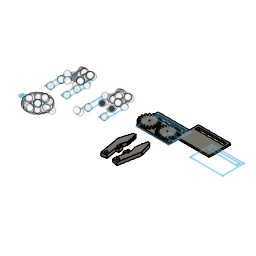
Garra-GSMAKERLAB (Autodesk Fusion 360 design; units mm, degrees)
part number: 2026-05-25-20-05-07-286
Autodesk Fusion 360 part; units mm, degrees
(part 1 of 2)
sketch "Esboço1" plane through (0, 0, 0) normal (0, 1, 0) x (1, 0, 0)
  line L0 (16, 125) -> (21, 125)
  line L1 (21, 103) -> (11, 103)
  line L2 (11, 103) -> (11, 125)
  line L3 (25, 125) -> (30, 125)
  line L4 (35, 125) -> (35, 103)
  line L5 (30, 103) -> (25, 103)
  line L6 (16, 108.5) -> (16, 125) construction
  line L7 (16, 114) -> (21, 114) construction
  line L8 (16, 114) -> (21, 114)
  line L9 (16, 119.5) -> (16, 125) construction
  line L10 (11, 119.5) -> (10, 119.5) construction
  line L11 (10, 119.5) -> (11, 119.5) construction
  line L12 (16, 119.5) -> (21, 119.5) construction
  line L13 (16, 103) -> (16, 114) construction
  line L14 (16, 108.5) -> (21, 108.5) construction
  line L15 (16, 108.5) -> (21, 108.5)
  line L16 (16, 108.5) -> (16, 114)
  line L17 (16, 119.5) -> (21, 119.5)
  line L18 (16, 119.5) -> (16, 125)
  line L19 (25, 114) -> (30, 114) construction
  line L20 (25, 114) -> (30, 114)
  line L21 (25, 119.5) -> (25, 125) construction
  line L22 (25, 119.5) -> (30, 119.5) construction
  line L23 (25, 114) -> (25, 108.5) construction
  line L24 (25, 108.5) -> (30, 108.5) construction
  line L25 (25, 108.5) -> (30, 108.5) construction
  line L26 (25, 108.5) -> (30, 108.5)
  line L27 (25, 119.5) -> (30, 119.5)
  line L28 (25, 108.5) -> (25, 114)
  line L29 (25, 119.5) -> (25, 125)
  line L30 (21, 119.5) -> (21, 114)
  line L31 (11, 103) -> (11, 100)
  line L32 (11, 100) -> (16, 100)
  line L33 (25, 103) -> (25, 100)
  line L34 (25, 100) -> (35, 100)
  line L35 (35, 100) -> (35, 103)
  line L36 (11, 125) -> (11, 127)
  line L37 (11, 127) -> (21, 127)
  line L38 (21, 127) -> (21, 125)
  line L39 (30, 127) -> (35, 127)
  line L40 (35, 125) -> (35, 127)
  line L41 (21, 108.5) -> (21, 103)
  line L42 (16, 103) -> (16, 100)
  line L43 (30, 125) -> (30, 127)
  line L44 (30, 103) -> (30, 108.5)
  line L45 (30, 114) -> (30, 119.5)
  arc A0 (237.1086, 129.0251) -> (213.2904, 133.6785) centre (216.5857, 87.2619) ccw
  arc A1 (237.2082, 125) -> (237.1086, 129.0251) centre (155.7746, 125) ccw
  arc A2 (213.2904, 116.3215) -> (237.1086, 120.9749) centre (216.5857, 162.7381) ccw
  arc A3 (237.1086, 120.9749) -> (237.2082, 125) centre (155.7746, 125) ccw
  arc A4 (230.8269, 156.6003) -> (206.8535, 152.8267) centre (225.8255, 110.3364) ccw
  arc A5 (212.79, 136.5164) -> (233.5803, 149.0355) centre (200.0111, 181.2609) ccw
  arc A6 (233.5803, 149.0355) -> (232.2971, 152.8519) centre (155.7746, 125) ccw
  arc A7 (232.2971, 152.8519) -> (230.8269, 156.6003) centre (155.7746, 125) ccw
  arc A8 (215.4928, 180.3639) -> (194.2558, 168.6185) centre (226.6162, 135.1795) ccw
  arc A9 (205.4127, 155.3223) -> (220.6674, 174.1971) centre (178.101, 192.9977) ccw
  arc A10 (220.6674, 174.1971) -> (218.1563, 177.3445) centre (155.7746, 125) ccw
  arc A11 (218.1563, 177.3445) -> (215.4928, 180.3639) centre (155.7746, 125) ccw
  arc A12 (192.9557, 197.4499) -> (177.0167, 179.1494) centre (218.8623, 158.7949) ccw
  arc A13 (192.0483, 170.4709) -> (199.9275, 193.4248) centre (153.4979, 196.533) ccw
  arc A14 (199.9275, 193.4248) -> (196.4914, 195.5235) centre (155.7746, 125) ccw
  arc A15 (196.4914, 195.5235) -> (192.9557, 197.4499) centre (155.7746, 125) ccw
  arc A16 (165.9341, 205.7973) -> (157.2155, 183.149) centre (203.4991, 178.3341) ccw
  arc A17 (174.3087, 180.135) -> (173.8621, 204.3994) centre (129.1695, 191.4404) ccw
  arc A18 (173.8621, 204.3994) -> (169.9154, 205.1964) centre (155.7746, 125) ccw
  arc A19 (169.9154, 205.1964) -> (165.9341, 205.7973) centre (155.7746, 125) ccw
  arc A20 (137.6871, 204.3994) -> (137.2404, 180.135) centre (182.3797, 191.4404) ccw
  arc A21 (154.3337, 183.149) -> (145.6151, 205.7973) centre (108.05, 178.3341) ccw
  arc A22 (145.6151, 205.7973) -> (141.6338, 205.1964) centre (155.7746, 125) ccw
  arc A23 (141.6338, 205.1964) -> (137.6871, 204.3994) centre (155.7746, 125) ccw
  arc A24 (111.6217, 193.4248) -> (119.5009, 170.4709) centre (158.0512, 196.533) ccw
  arc A25 (134.5325, 179.1494) -> (118.5935, 197.4499) centre (92.6869, 158.7949) ccw
  arc A26 (118.5935, 197.4499) -> (115.0578, 195.5235) centre (155.7746, 125) ccw
  arc A27 (115.0578, 195.5235) -> (111.6217, 193.4248) centre (155.7746, 125) ccw
  arc A28 (90.8818, 174.1971) -> (106.1365, 155.3223) centre (133.4482, 192.9977) ccw
  arc A29 (117.2934, 168.6185) -> (96.0564, 180.3639) centre (84.933, 135.1795) ccw
  arc A30 (96.0564, 180.3639) -> (93.3929, 177.3445) centre (155.7746, 125) ccw
  arc A31 (93.3929, 177.3445) -> (90.8818, 174.1971) centre (155.7746, 125) ccw
  arc A32 (77.9689, 149.0355) -> (98.7592, 136.5164) centre (111.5381, 181.2609) ccw
  arc A33 (104.6957, 152.8267) -> (80.7223, 156.6003) centre (85.7237, 110.3364) ccw
  arc A34 (80.7223, 156.6003) -> (79.2521, 152.8519) centre (155.7746, 125) ccw
  arc A35 (79.2521, 152.8519) -> (77.9689, 149.0355) centre (155.7746, 125) ccw
  arc A36 (74.4406, 120.9749) -> (98.2588, 116.3215) centre (94.9635, 162.7381) ccw
  arc A37 (98.2588, 133.6785) -> (74.4406, 129.0251) centre (94.9635, 87.2619) ccw
  arc A38 (74.4406, 129.0251) -> (74.341, 125) centre (155.7746, 125) ccw
  arc A39 (74.341, 125) -> (74.4406, 120.9749) centre (155.7746, 125) ccw
  arc A40 (80.7223, 93.3997) -> (104.6957, 97.1733) centre (85.7237, 139.6636) ccw
  arc A41 (98.7592, 113.4836) -> (77.9689, 100.9645) centre (111.5381, 68.7391) ccw
  arc A42 (77.9689, 100.9645) -> (79.2521, 97.1481) centre (155.7746, 125) ccw
  arc A43 (79.2521, 97.1481) -> (80.7223, 93.3997) centre (155.7746, 125) ccw
  arc A44 (96.0564, 69.6361) -> (117.2934, 81.3815) centre (84.933, 114.8205) ccw
  arc A45 (106.1365, 94.6777) -> (90.8818, 75.8029) centre (133.4482, 57.0023) ccw
  arc A46 (90.8818, 75.8029) -> (93.3929, 72.6555) centre (155.7746, 125) ccw
  arc A47 (93.3929, 72.6555) -> (96.0564, 69.6361) centre (155.7746, 125) ccw
  arc A48 (118.5935, 52.5501) -> (134.5325, 70.8506) centre (92.6869, 91.2051) ccw
  arc A49 (119.5009, 79.5291) -> (111.6217, 56.5752) centre (158.0512, 53.467) ccw
  arc A50 (111.6217, 56.5752) -> (115.0578, 54.4765) centre (155.7746, 125) ccw
  arc A51 (115.0578, 54.4765) -> (118.5935, 52.5501) centre (155.7746, 125) ccw
  arc A52 (145.6151, 44.2027) -> (154.3337, 66.851) centre (108.05, 71.6659) ccw
  arc A53 (137.2404, 69.865) -> (137.6871, 45.6006) centre (182.3797, 58.5596) ccw
  arc A54 (137.6871, 45.6006) -> (141.6338, 44.8036) centre (155.7746, 125) ccw
  arc A55 (141.6338, 44.8036) -> (145.6151, 44.2027) centre (155.7746, 125) ccw
  arc A56 (173.8621, 45.6006) -> (174.3087, 69.865) centre (129.1695, 58.5596) ccw
  arc A57 (157.2155, 66.851) -> (165.9341, 44.2027) centre (203.4991, 71.6659) ccw
  arc A58 (165.9341, 44.2027) -> (169.9154, 44.8036) centre (155.7746, 125) ccw
  arc A59 (169.9154, 44.8036) -> (173.8621, 45.6006) centre (155.7746, 125) ccw
  arc A60 (199.9275, 56.5752) -> (192.0483, 79.5291) centre (153.4979, 53.467) ccw
  arc A61 (177.0167, 70.8506) -> (192.9557, 52.5501) centre (218.8623, 91.2051) ccw
  arc A62 (192.9557, 52.5501) -> (196.4914, 54.4765) centre (155.7746, 125) ccw
  arc A63 (196.4914, 54.4765) -> (199.9275, 56.5752) centre (155.7746, 125) ccw
  arc A64 (220.6674, 75.8029) -> (205.4127, 94.6777) centre (178.101, 57.0023) ccw
  arc A65 (194.2558, 81.3815) -> (215.4928, 69.6361) centre (226.6162, 114.8205) ccw
  arc A66 (215.4928, 69.6361) -> (218.1563, 72.6555) centre (155.7746, 125) ccw
  arc A67 (218.1563, 72.6555) -> (220.6674, 75.8029) centre (155.7746, 125) ccw
  arc A68 (233.5803, 100.9645) -> (212.79, 113.4836) centre (200.0111, 68.7391) ccw
  arc A69 (206.8535, 97.1733) -> (230.8269, 93.3997) centre (225.8255, 139.6636) ccw
  arc A70 (230.8269, 93.3997) -> (232.2971, 97.1481) centre (155.7746, 125) ccw
  arc A71 (232.2971, 97.1481) -> (233.5803, 100.9645) centre (155.7746, 125) ccw
  arc A72 (106.1365, 155.3223) -> (104.6957, 152.8267) centre (155.7746, 125) ccw
  arc A73 (119.5009, 170.4709) -> (117.2934, 168.6185) centre (155.7746, 125) ccw
  arc A74 (137.2404, 180.135) -> (134.5325, 179.1494) centre (155.7746, 125) ccw
  arc A75 (157.2155, 183.149) -> (154.3337, 183.149) centre (155.7746, 125) ccw
  arc A76 (177.0167, 179.1494) -> (174.3087, 180.135) centre (155.7746, 125) ccw
  arc A77 (194.2558, 168.6185) -> (192.0483, 170.4709) centre (155.7746, 125) ccw
  arc A78 (206.8535, 152.8267) -> (205.4127, 155.3223) centre (155.7746, 125) ccw
  arc A79 (213.2904, 133.6785) -> (212.79, 136.5164) centre (155.7746, 125) ccw
  arc A80 (212.79, 113.4836) -> (213.2904, 116.3215) centre (155.7746, 125) ccw
  arc A81 (205.4127, 94.6777) -> (206.8535, 97.1733) centre (155.7746, 125) ccw
  arc A82 (192.0483, 79.5291) -> (194.2558, 81.3815) centre (155.7746, 125) ccw
  arc A83 (174.3087, 69.865) -> (177.0167, 70.8506) centre (155.7746, 125) ccw
  arc A84 (154.3337, 66.851) -> (157.2155, 66.851) centre (155.7746, 125) ccw
  arc A85 (134.5325, 70.8506) -> (137.2404, 69.865) centre (155.7746, 125) ccw
  arc A86 (117.2934, 81.3815) -> (119.5009, 79.5291) centre (155.7746, 125) ccw
  arc A87 (104.6957, 97.1733) -> (106.1365, 94.6777) centre (155.7746, 125) ccw
  arc A88 (98.7592, 136.5164) -> (98.2588, 133.6785) centre (155.7746, 125) ccw
  arc A89 (98.2588, 116.3215) -> (98.7592, 113.4836) centre (155.7746, 125) ccw
  circle A90 centre (155.7746, 125) radius 5.4289
  line L46 (120, 600) -> (106.1803, 600)
  arc A91 (106.1803, 600) -> (96.5303, 592.6223) centre (106.1803, 590) ccw
  circle A92 centre (75, 425) radius 12.5
  line L47 (50, 497.6393) -> (50, 450)
  line L48 (50, 450) -> (50, 400)
  line L49 (101.0557, 452.1115) -> (123.4164, 496.8328)
  arc A93 (51.0557, 502.1115) -> (50, 497.6393) centre (60, 497.6393) ccw
  arc A94 (106.1803, 600) -> (97.2361, 594.4721) centre (106.1803, 590) ccw
  line L50 (51.0557, 502.1115) -> (97.2361, 594.4721)
  arc A95 (123.4164, 496.8328) -> (124.5987, 500.0947) centre (110, 503.541) ccw
  line L51 (100, 400) -> (100, 447.6393)
  arc A96 (101.0557, 452.1115) -> (100, 447.6393) centre (110, 447.6393) ccw
  line L52 (120, 600) -> (106.1803, 600)
  circle A97 centre (75, 425) radius 12.5
  line L53 (250, 400) -> (250, 497.732)
  line L54 (200, 400) -> (200, 446.5033)
  line L55 (198.9884, 450.8862) -> (176.5174, 496.9698)
  line L56 (180, 600) -> (196.9111, 600)
  line L57 (201.3824, 597.2378) -> (248.9426, 502.2076)
  arc A98 (200, 446.5033) -> (198.9884, 450.8862) centre (190, 446.5033) ccw
  arc A99 (175.3938, 500.1297) -> (176.5174, 496.9698) centre (190, 503.544) ccw
  arc A100 (180, 600) -> (175.3489, 596.8351) centre (180, 595) ccw
  arc A101 (124.6389, 596.8655) -> (120, 600) centre (120, 595) ccw
  arc A102 (201.3824, 597.2378) -> (196.9111, 600) centre (196.9111, 595) ccw
  arc A103 (250, 497.732) -> (248.9426, 502.2076) centre (240, 497.732) ccw
  circle A104 centre (225, 423.2517) radius 12.5
  arc A105 (125, 510.1754) -> (125, 505.1805) centre (124.8879, 507.678) ccw
  line L58 (125, 505.0754) -> (125, 505.1805)
  line L59 (125, 505.0754) -> (125, 505.1805)
  arc A106 (125, 520.3754) -> (125, 515.3805) centre (124.8879, 517.878) ccw
  arc A107 (125, 530.5754) -> (125, 525.5805) centre (124.8879, 528.078) ccw
  arc A108 (125, 540.7754) -> (125, 535.7805) centre (124.8879, 538.278) ccw
  arc A109 (125, 550.9754) -> (125, 545.9805) centre (124.8879, 548.478) ccw
  arc A110 (125, 561.1754) -> (125, 556.1805) centre (124.8879, 558.678) ccw
  arc A111 (125, 571.3754) -> (125, 566.3805) centre (124.8879, 568.878) ccw
  arc A112 (125, 581.5754) -> (125, 576.5805) centre (124.8879, 579.078) ccw
  arc A113 (125, 591.7754) -> (125, 586.7805) centre (124.8879, 589.278) ccw
  line L60 (125, 591.7754) -> (125, 591.8805)
  line L61 (125, 591.7754) -> (125, 591.8805)
  arc A114 (175, 510.2805) -> (175, 515.2754) centre (174.8879, 512.778) ccw
  arc A115 (175, 520.4805) -> (175, 525.4754) centre (174.8879, 522.978) ccw
  arc A116 (175, 530.6805) -> (175, 535.6754) centre (174.8879, 533.178) ccw
  arc A117 (175, 540.8805) -> (175, 545.8754) centre (174.8879, 543.378) ccw
  arc A118 (175, 551.0805) -> (175, 556.0754) centre (174.8879, 553.578) ccw
  arc A119 (175, 561.2805) -> (175, 566.2754) centre (174.8879, 563.778) ccw
  arc A120 (175, 571.4805) -> (175, 576.4754) centre (174.8879, 573.978) ccw
  arc A121 (175, 581.6805) -> (175, 586.6754) centre (174.8879, 584.178) ccw
  arc A122 (175, 591.8805) -> (175.3489, 596.8351) centre (174.8879, 594.378) ccw
  arc A123 (124.5987, 500.0947) -> (125, 505.0754) centre (124.8879, 502.578) ccw
  arc A124 (125, 510.2805) -> (125, 515.2754) centre (124.8879, 512.778) ccw
  line L62 (125, 510.1754) -> (125, 510.2805)
  line L63 (125, 515.2754) -> (125, 515.3805)
  line L64 (125, 510.1754) -> (125, 510.2805)
  line L65 (125, 515.2754) -> (125, 515.3805)
  arc A125 (125, 520.4805) -> (125, 525.4754) centre (124.8879, 522.978) ccw
  line L66 (125, 520.3754) -> (125, 520.4805)
  line L67 (125, 525.4754) -> (125, 525.5805)
  line L68 (125, 520.3754) -> (125, 520.4805)
  line L69 (125, 525.4754) -> (125, 525.5805)
  arc A126 (125, 530.6805) -> (125, 535.6754) centre (124.8879, 533.178) ccw
  line L70 (125, 530.5754) -> (125, 530.6805)
  line L71 (125, 535.6754) -> (125, 535.7805)
  line L72 (125, 530.5754) -> (125, 530.6805)
  line L73 (125, 535.6754) -> (125, 535.7805)
  arc A127 (125, 540.8805) -> (125, 545.8754) centre (124.8879, 543.378) ccw
  line L74 (125, 540.7754) -> (125, 540.8805)
  line L75 (125, 545.8754) -> (125, 545.9805)
  line L76 (125, 540.7754) -> (125, 540.8805)
  line L77 (125, 545.8754) -> (125, 545.9805)
  arc A128 (125, 551.0805) -> (125, 556.0754) centre (124.8879, 553.578) ccw
  line L78 (125, 550.9754) -> (125, 551.0805)
  line L79 (125, 556.0754) -> (125, 556.1805)
  line L80 (125, 550.9754) -> (125, 551.0805)
  line L81 (125, 556.0754) -> (125, 556.1805)
  arc A129 (125, 561.2805) -> (125, 566.2754) centre (124.8879, 563.778) ccw
  line L82 (125, 561.1754) -> (125, 561.2805)
  line L83 (125, 566.2754) -> (125, 566.3805)
  line L84 (125, 561.1754) -> (125, 561.2805)
  line L85 (125, 566.2754) -> (125, 566.3805)
  arc A130 (125, 571.4805) -> (125, 576.4754) centre (124.8879, 573.978) ccw
  line L86 (125, 571.3754) -> (125, 571.4805)
  line L87 (125, 576.4754) -> (125, 576.5805)
  line L88 (125, 571.3754) -> (125, 571.4805)
  line L89 (125, 576.4754) -> (125, 576.5805)
  arc A131 (125, 581.6805) -> (125, 586.6754) centre (124.8879, 584.178) ccw
  line L90 (125, 581.5754) -> (125, 581.6805)
  line L91 (125, 586.6754) -> (125, 586.7805)
  line L92 (125, 581.5754) -> (125, 581.6805)
  line L93 (125, 586.6754) -> (125, 586.7805)
  arc A132 (125, 591.8805) -> (124.6389, 596.8655) centre (124.8879, 594.378) ccw
  arc A133 (175, 510.1754) -> (175, 505.1805) centre (174.8879, 507.678) ccw
  line L94 (175, 505.0754) -> (175, 505.1805)
  line L95 (175, 510.1754) -> (175, 510.2805)
  arc A134 (175, 520.3754) -> (175, 515.3805) centre (174.8879, 517.878) ccw
  line L96 (175, 515.2754) -> (175, 515.3805)
  line L97 (175, 520.3754) -> (175, 520.4805)
  arc A135 (175, 530.5754) -> (175, 525.5805) centre (174.8879, 528.078) ccw
  line L98 (175, 525.4754) -> (175, 525.5805)
  line L99 (175, 530.5754) -> (175, 530.6805)
  arc A136 (175, 540.7754) -> (175, 535.7805) centre (174.8879, 538.278) ccw
  line L100 (175, 535.6754) -> (175, 535.7805)
  line L101 (175, 540.7754) -> (175, 540.8805)
  arc A137 (175, 550.9754) -> (175, 545.9805) centre (174.8879, 548.478) ccw
  line L102 (175, 545.8754) -> (175, 545.9805)
  line L103 (175, 550.9754) -> (175, 551.0805)
  arc A138 (175, 561.1754) -> (175, 556.1805) centre (174.8879, 558.678) ccw
  line L104 (175, 556.0754) -> (175, 556.1805)
  line L105 (175, 561.1754) -> (175, 561.2805)
  arc A139 (175, 571.3754) -> (175, 566.3805) centre (174.8879, 568.878) ccw
  line L106 (175, 566.2754) -> (175, 566.3805)
  line L107 (175, 571.3754) -> (175, 571.4805)
  arc A140 (175, 581.5754) -> (175, 576.5805) centre (174.8879, 579.078) ccw
  line L108 (175, 576.4754) -> (175, 576.5805)
  line L109 (175, 581.5754) -> (175, 581.6805)
  arc A141 (175, 591.7754) -> (175, 586.7805) centre (174.8879, 589.278) ccw
  line L110 (175, 586.6754) -> (175, 586.7805)
  line L111 (175, 591.7754) -> (175, 591.8805)
  arc A142 (175.3938, 500.1297) -> (175, 505.0754) centre (174.8879, 502.578) ccw
  line L112 (50, 400) -> (50, 300)
  line L113 (50, 300) -> (100, 300)
  line L114 (100, 300) -> (100, 400)
  line L115 (200, 400) -> (200, 300)
  line L116 (200, 300) -> (250, 300)
  line L117 (250, 300) -> (250, 400)
  circle A143 centre (75, 325) radius 12.5
  circle A144 centre (225, 325) radius 12.5
  circle A145 centre (251, 128) radius 7.2111
  circle A146 centre (281, 133) radius 10.5
  line L118 (100, 300) -> (125, 300) construction
  line L119 (125, 300) -> (125, 250) construction
  line L120 (125, 250) -> (45, 250) construction
  line L121 (45, 250) -> (45, 300) construction
  line L122 (45, 300) -> (50, 300) construction
  line L123 (100, 300) -> (125, 250) construction
  line L124 (50, 300) -> (75, 250) construction
  line L125 (800, 600) -> (1100, 600)
  line L126 (1100, 600) -> (1100, 400)
  line L127 (1100, 400) -> (800, 400)
  line L128 (800, 400) -> (800, 600)
  line L129 (1000, 500) -> (1090, 500)
  line L130 (1090, 500) -> (1090, 450)
  line L131 (1090, 450) -> (1000, 450)
  line L132 (1000, 450) -> (1000, 500)
  line L133 (820, 580) -> (1080, 580)
  line L134 (1080, 580) -> (1080, 550)
  line L135 (1080, 550) -> (820, 550)
  line L136 (820, 550) -> (820, 580)
  arc A147 (104.6957, 152.8267) -> (80.7223, 156.6003) centre (85.7237, 110.3364) ccw
  arc A148 (232.2971, 152.8519) -> (230.8269, 156.6003) centre (155.7746, 125) ccw
  arc A149 (141.6338, 205.1964) -> (137.6871, 204.3994) centre (155.7746, 125) ccw
  arc A150 (206.8535, 152.8267) -> (205.4127, 155.3223) centre (155.7746, 125) ccw
  arc A151 (230.8269, 156.6003) -> (206.8535, 152.8267) centre (225.8255, 110.3364) ccw
  arc A152 (80.7223, 156.6003) -> (79.2521, 152.8519) centre (155.7746, 125) ccw
  arc A153 (154.3337, 183.149) -> (145.6151, 205.7973) centre (108.05, 178.3341) ccw
  arc A154 (145.6151, 205.7973) -> (141.6338, 205.1964) centre (155.7746, 125) ccw
  arc A155 (137.6871, 204.3994) -> (137.2404, 180.135) centre (182.3797, 191.4404) ccw
  arc A156 (220.6674, 75.8029) -> (205.4127, 94.6777) centre (178.101, 57.0023) ccw
  arc A157 (194.2558, 81.3815) -> (215.4928, 69.6361) centre (226.6162, 114.8205) ccw
  arc A158 (104.6957, 97.1733) -> (106.1365, 94.6777) centre (155.7746, 125) ccw
  arc A159 (169.9154, 44.8036) -> (173.8621, 45.6006) centre (155.7746, 125) ccw
  arc A160 (232.2971, 97.1481) -> (233.5803, 100.9645) centre (155.7746, 125) ccw
  arc A161 (118.5935, 52.5501) -> (134.5325, 70.8506) centre (92.6869, 91.2051) ccw
  arc A162 (90.8818, 75.8029) -> (93.3929, 72.6555) centre (155.7746, 125) ccw
  arc A163 (218.1563, 72.6555) -> (220.6674, 75.8029) centre (155.7746, 125) ccw
  arc A164 (174.3087, 69.865) -> (177.0167, 70.8506) centre (155.7746, 125) ccw
  arc A165 (206.8535, 97.1733) -> (230.8269, 93.3997) centre (225.8255, 139.6636) ccw
  arc A166 (137.6871, 45.6006) -> (141.6338, 44.8036) centre (155.7746, 125) ccw
  arc A167 (165.9341, 44.2027) -> (169.9154, 44.8036) centre (155.7746, 125) ccw
  arc A168 (137.2404, 69.865) -> (137.6871, 45.6006) centre (182.3797, 58.5596) ccw
  arc A169 (111.6217, 56.5752) -> (115.0578, 54.4765) centre (155.7746, 125) ccw
  arc A170 (117.2934, 81.3815) -> (119.5009, 79.5291) centre (155.7746, 125) ccw
  arc A171 (145.6151, 44.2027) -> (154.3337, 66.851) centre (108.05, 71.6659) ccw
  arc A172 (93.3929, 72.6555) -> (96.0564, 69.6361) centre (155.7746, 125) ccw
  arc A173 (134.5325, 70.8506) -> (137.2404, 69.865) centre (155.7746, 125) ccw
  arc A174 (215.4928, 69.6361) -> (218.1563, 72.6555) centre (155.7746, 125) ccw
  arc A175 (199.9275, 56.5752) -> (192.0483, 79.5291) centre (153.4979, 53.467) ccw
  arc A176 (173.8621, 45.6006) -> (174.3087, 69.865) centre (129.1695, 58.5596) ccw
  arc A177 (141.6338, 44.8036) -> (145.6151, 44.2027) centre (155.7746, 125) ccw
  arc A178 (192.9557, 52.5501) -> (196.4914, 54.4765) centre (155.7746, 125) ccw
  arc A179 (106.1365, 94.6777) -> (90.8818, 75.8029) centre (133.4482, 57.0023) ccw
  arc A180 (230.8269, 93.3997) -> (232.2971, 97.1481) centre (155.7746, 125) ccw
  arc A181 (196.4914, 54.4765) -> (199.9275, 56.5752) centre (155.7746, 125) ccw
  arc A182 (177.0167, 70.8506) -> (192.9557, 52.5501) centre (218.8623, 91.2051) ccw
  arc A183 (192.0483, 79.5291) -> (194.2558, 81.3815) centre (155.7746, 125) ccw
  arc A184 (119.5009, 79.5291) -> (111.6217, 56.5752) centre (158.0512, 53.467) ccw
  arc A185 (117.2934, 168.6185) -> (96.0564, 180.3639) centre (84.933, 135.1795) ccw
  arc A186 (115.0578, 195.5235) -> (111.6217, 193.4248) centre (155.7746, 125) ccw
  arc A187 (111.6217, 193.4248) -> (119.5009, 170.4709) centre (158.0512, 196.533) ccw
  arc A188 (137.2404, 180.135) -> (134.5325, 179.1494) centre (155.7746, 125) ccw
  arc A189 (218.1563, 177.3445) -> (215.4928, 180.3639) centre (155.7746, 125) ccw
  circle A190 centre (155.7746, 125) radius 5.4289
  arc A191 (174.3087, 180.135) -> (173.8621, 204.3994) centre (129.1695, 191.4404) ccw
  arc A192 (77.9689, 149.0355) -> (98.7592, 136.5164) centre (111.5381, 181.2609) ccw
  arc A193 (74.4406, 120.9749) -> (98.2588, 116.3215) centre (94.9635, 162.7381) ccw
  arc A194 (192.0483, 170.4709) -> (199.9275, 193.4248) centre (153.4979, 196.533) ccw
  arc A195 (74.4406, 129.0251) -> (74.341, 125) centre (155.7746, 125) ccw
  arc A196 (74.341, 125) -> (74.4406, 120.9749) centre (155.7746, 125) ccw
  arc A197 (205.4127, 155.3223) -> (220.6674, 174.1971) centre (178.101, 192.9977) ccw
  arc A198 (199.9275, 193.4248) -> (196.4914, 195.5235) centre (155.7746, 125) ccw
  arc A199 (173.8621, 204.3994) -> (169.9154, 205.1964) centre (155.7746, 125) ccw
  arc A200 (79.2521, 152.8519) -> (77.9689, 149.0355) centre (155.7746, 125) ccw
  arc A201 (194.2558, 168.6185) -> (192.0483, 170.4709) centre (155.7746, 125) ccw
  arc A202 (215.4928, 180.3639) -> (194.2558, 168.6185) centre (226.6162, 135.1795) ccw
  arc A203 (233.5803, 149.0355) -> (232.2971, 152.8519) centre (155.7746, 125) ccw
  arc A204 (237.1086, 129.0251) -> (213.2904, 133.6785) centre (216.5857, 87.2619) ccw
  arc A205 (237.2082, 125) -> (237.1086, 129.0251) centre (155.7746, 125) ccw
  arc A206 (98.2588, 133.6785) -> (74.4406, 129.0251) centre (94.9635, 87.2619) ccw
  arc A207 (154.3337, 66.851) -> (157.2155, 66.851) centre (155.7746, 125) ccw
  arc A208 (98.7592, 136.5164) -> (98.2588, 133.6785) centre (155.7746, 125) ccw
  arc A209 (213.2904, 133.6785) -> (212.79, 136.5164) centre (155.7746, 125) ccw
  arc A210 (212.79, 136.5164) -> (233.5803, 149.0355) centre (200.0111, 181.2609) ccw
  arc A211 (177.0167, 179.1494) -> (174.3087, 180.135) centre (155.7746, 125) ccw
  arc A212 (212.79, 113.4836) -> (213.2904, 116.3215) centre (155.7746, 125) ccw
  arc A213 (169.9154, 205.1964) -> (165.9341, 205.7973) centre (155.7746, 125) ccw
  arc A214 (196.4914, 195.5235) -> (192.9557, 197.4499) centre (155.7746, 125) ccw
  arc A215 (165.9341, 205.7973) -> (157.2155, 183.149) centre (203.4991, 178.3341) ccw
  arc A216 (213.2904, 116.3215) -> (237.1086, 120.9749) centre (216.5857, 162.7381) ccw
  arc A217 (205.4127, 94.6777) -> (206.8535, 97.1733) centre (155.7746, 125) ccw
  arc A218 (98.2588, 116.3215) -> (98.7592, 113.4836) centre (155.7746, 125) ccw
  arc A219 (98.7592, 113.4836) -> (77.9689, 100.9645) centre (111.5381, 68.7391) ccw
  arc A220 (77.9689, 100.9645) -> (79.2521, 97.1481) centre (155.7746, 125) ccw
  arc A221 (237.1086, 120.9749) -> (237.2082, 125) centre (155.7746, 125) ccw
  arc A222 (80.7223, 93.3997) -> (104.6957, 97.1733) centre (85.7237, 139.6636) ccw
  arc A223 (220.6674, 174.1971) -> (218.1563, 177.3445) centre (155.7746, 125) ccw
  arc A224 (157.2155, 183.149) -> (154.3337, 183.149) centre (155.7746, 125) ccw
  arc A225 (233.5803, 100.9645) -> (212.79, 113.4836) centre (200.0111, 68.7391) ccw
  arc A226 (157.2155, 66.851) -> (165.9341, 44.2027) centre (203.4991, 71.6659) ccw
  arc A227 (192.9557, 197.4499) -> (177.0167, 179.1494) centre (218.8623, 158.7949) ccw
  arc A228 (90.8818, 174.1971) -> (106.1365, 155.3223) centre (133.4482, 192.9977) ccw
  arc A229 (96.0564, 180.3639) -> (93.3929, 177.3445) centre (155.7746, 125) ccw
  arc A230 (106.1365, 155.3223) -> (104.6957, 152.8267) centre (155.7746, 125) ccw
  arc A231 (93.3929, 177.3445) -> (90.8818, 174.1971) centre (155.7746, 125) ccw
  arc A232 (134.5325, 179.1494) -> (118.5935, 197.4499) centre (92.6869, 158.7949) ccw
  arc A233 (118.5935, 197.4499) -> (115.0578, 195.5235) centre (155.7746, 125) ccw
  arc A234 (119.5009, 170.4709) -> (117.2934, 168.6185) centre (155.7746, 125) ccw
  arc A235 (96.0564, 69.6361) -> (117.2934, 81.3815) centre (84.933, 114.8205) ccw
  arc A236 (79.2521, 97.1481) -> (80.7223, 93.3997) centre (155.7746, 125) ccw
  arc A237 (115.0578, 54.4765) -> (118.5935, 52.5501) centre (155.7746, 125) ccw
  line L137 (100, 445) -> (200, 445) construction
  line L138 (100, 400) -> (200, 400) construction
  line L139 (150, 445) -> (150, 400) construction
  line L140 (400, 450) -> (400, 400)
  line L141 (450, 400) -> (550, 400) construction
  line L142 (600, 300) -> (600, 400)
  arc A238 (600, 497.732) -> (598.9426, 502.2076) centre (590, 497.732) ccw
  line L143 (600, 400) -> (600, 497.732)
  arc A239 (525, 581.5754) -> (525, 576.5805) centre (524.8879, 579.078) ccw
  arc A240 (525, 520.3754) -> (525, 515.3805) centre (524.8879, 517.878) ccw
  line L144 (525, 581.5754) -> (525, 581.6805)
  line L145 (525, 576.4754) -> (525, 576.5805)
  arc A241 (401.0557, 502.1115) -> (400, 497.6393) centre (410, 497.6393) ccw
  line L146 (525, 545.8754) -> (525, 545.9805)
  arc A242 (475, 540.7754) -> (475, 535.7805) centre (474.8879, 538.278) ccw
  arc A243 (475, 510.2805) -> (475, 515.2754) centre (474.8879, 512.778) ccw
  arc A244 (530, 600) -> (525.3489, 596.8351) centre (530, 595) ccw
  line L147 (475, 550.9754) -> (475, 551.0805)
  line L148 (525, 510.1754) -> (525, 510.2805)
  arc A245 (525.3938, 500.1297) -> (525, 505.0754) centre (524.8879, 502.578) ccw
  line L149 (525, 520.3754) -> (525, 520.4805)
  arc A246 (475, 520.3754) -> (475, 515.3805) centre (474.8879, 517.878) ccw
  line L150 (475, 505.0754) -> (475, 505.1805)
  arc A247 (525.3938, 500.1297) -> (526.5174, 496.9698) centre (540, 503.544) ccw
  arc A248 (525, 510.1754) -> (525, 505.1805) centre (524.8879, 507.678) ccw
  arc A249 (525, 591.7754) -> (525, 586.7805) centre (524.8879, 589.278) ccw
  line L151 (475, 591.7754) -> (475, 591.8805)
  line L152 (525, 525.4754) -> (525, 525.5805)
  arc A250 (456.1803, 600) -> (447.2361, 594.4721) centre (456.1803, 590) ccw
  line L153 (475, 545.8754) -> (475, 545.9805)
  line L154 (475, 530.5754) -> (475, 530.6805)
  arc A251 (551.3824, 597.2378) -> (546.9111, 600) centre (546.9111, 595) ccw
  line L155 (475, 520.3754) -> (475, 520.4805)
  line L156 (475, 510.1754) -> (475, 510.2805)
  line L157 (525, 535.6754) -> (525, 535.7805)
  arc A252 (525, 540.8805) -> (525, 545.8754) centre (524.8879, 543.378) ccw
  line L158 (475, 571.3754) -> (475, 571.4805)
  line L159 (475, 545.8754) -> (475, 545.9805)
  line L160 (475, 515.2754) -> (475, 515.3805)
  line L161 (401.0557, 502.1115) -> (447.2361, 594.4721)
  line L162 (525, 530.5754) -> (525, 530.6805)
  arc A253 (475, 550.9754) -> (475, 545.9805) centre (474.8879, 548.478) ccw
  arc A254 (475, 510.1754) -> (475, 505.1805) centre (474.8879, 507.678) ccw
  line L163 (475, 535.6754) -> (475, 535.7805)
  arc A255 (525, 581.6805) -> (525, 586.6754) centre (524.8879, 584.178) ccw
  line L164 (525, 540.7754) -> (525, 540.8805)
  line L165 (400, 400) -> (400, 300)
  arc A256 (525, 540.7754) -> (525, 535.7805) centre (524.8879, 538.278) ccw
  line L166 (450, 300) -> (450, 400)
  line L167 (525, 556.0754) -> (525, 556.1805)
  line L168 (450, 300) -> (475, 250) construction
  line L169 (450, 300) -> (475, 300) construction
  line L170 (525, 571.3754) -> (525, 571.4805)
  line L171 (525, 515.2754) -> (525, 515.3805)
  arc A257 (525, 561.1754) -> (525, 556.1805) centre (524.8879, 558.678) ccw
  arc A258 (525, 530.5754) -> (525, 525.5805) centre (524.8879, 528.078) ccw
  line L172 (525, 561.1754) -> (525, 561.2805)
  arc A259 (525, 520.4805) -> (525, 525.4754) centre (524.8879, 522.978) ccw
  line L173 (550, 400) -> (550, 300)
  arc A260 (525, 571.4805) -> (525, 576.4754) centre (524.8879, 573.978) ccw
  arc A261 (525, 510.2805) -> (525, 515.2754) centre (524.8879, 512.778) ccw
  line L174 (470, 600) -> (456.1803, 600)
  arc A262 (456.1803, 600) -> (446.5303, 592.6223) centre (456.1803, 590) ccw
  line L175 (525, 505.0754) -> (525, 505.1805)
  arc A263 (525, 530.6805) -> (525, 535.6754) centre (524.8879, 533.178) ccw
  arc A264 (525, 571.3754) -> (525, 566.3805) centre (524.8879, 568.878) ccw
  arc A265 (525, 551.0805) -> (525, 556.0754) centre (524.8879, 553.578) ccw
  line L176 (525, 550.9754) -> (525, 551.0805)
  line L177 (475, 540.7754) -> (475, 540.8805)
  line L178 (525, 566.2754) -> (525, 566.3805)
  arc A266 (474.5987, 500.0947) -> (475, 505.0754) centre (474.8879, 502.578) ccw
  arc A267 (525, 561.2805) -> (525, 566.2754) centre (524.8879, 563.778) ccw
  arc A268 (475, 540.8805) -> (475, 545.8754) centre (474.8879, 543.378) ccw
  line L179 (475, 581.5754) -> (475, 581.6805)
  circle A269 centre (575, 325) radius 12.5
  line L180 (470, 600) -> (456.1803, 600)
  line L181 (451.0557, 452.1115) -> (473.4164, 496.8328)
  line L182 (550, 300) -> (600, 300)
  line L183 (400, 497.6393) -> (400, 450)
  line L184 (548.9884, 450.8862) -> (526.5174, 496.9698)
  circle A270 centre (425, 325) radius 12.5
  line L185 (450, 445) -> (550, 445) construction
  line L186 (475, 556.0754) -> (475, 556.1805)
  line L187 (475, 530.5754) -> (475, 530.6805)
  arc A271 (475, 581.5754) -> (475, 576.5805) centre (474.8879, 579.078) ccw
  arc A272 (475, 530.6805) -> (475, 535.6754) centre (474.8879, 533.178) ccw
  line L188 (525, 591.7754) -> (525, 591.8805)
  arc A273 (473.4164, 496.8328) -> (474.5987, 500.0947) centre (460, 503.541) ccw
  line L189 (475, 540.7754) -> (475, 540.8805)
  arc A274 (475, 561.1754) -> (475, 556.1805) centre (474.8879, 558.678) ccw
  arc A275 (475, 561.2805) -> (475, 566.2754) centre (474.8879, 563.778) ccw
  line L190 (525, 586.6754) -> (525, 586.7805)
  line L191 (475, 525.4754) -> (475, 525.5805)
  line L192 (475, 550.9754) -> (475, 551.0805)
  line L193 (475, 510.1754) -> (475, 510.2805)
  line L194 (475, 576.4754) -> (475, 576.5805)
  arc A276 (475, 530.5754) -> (475, 525.5805) centre (474.8879, 528.078) ccw
  arc A277 (525, 591.8805) -> (525.3489, 596.8351) centre (524.8879, 594.378) ccw
  arc A278 (475, 571.4805) -> (475, 576.4754) centre (474.8879, 573.978) ccw
  line L195 (530, 600) -> (546.9111, 600)
  line L196 (475, 556.0754) -> (475, 556.1805)
  line L197 (475, 535.6754) -> (475, 535.7805)
  line L198 (475, 515.2754) -> (475, 515.3805)
  line L199 (475, 586.6754) -> (475, 586.7805)
  arc A279 (474.6389, 596.8655) -> (470, 600) centre (470, 595) ccw
  line L200 (475, 591.7754) -> (475, 591.8805)
  line L201 (475, 561.1754) -> (475, 561.2805)
  arc A280 (475, 571.3754) -> (475, 566.3805) centre (474.8879, 568.878) ccw
  arc A281 (475, 591.7754) -> (475, 586.7805) centre (474.8879, 589.278) ccw
  line L202 (475, 561.1754) -> (475, 561.2805)
  line L203 (475, 566.2754) -> (475, 566.3805)
  line L204 (475, 571.3754) -> (475, 571.4805)
  line L205 (475, 520.3754) -> (475, 520.4805)
  line L206 (475, 566.2754) -> (475, 566.3805)
  line L207 (475, 581.5754) -> (475, 581.6805)
  line L208 (475, 586.6754) -> (475, 586.7805)
  line L209 (475, 525.4754) -> (475, 525.5805)
  line L210 (475, 576.4754) -> (475, 576.5805)
  arc A282 (475, 581.6805) -> (475, 586.6754) centre (474.8879, 584.178) ccw
  arc A283 (475, 591.8805) -> (474.6389, 596.8655) centre (474.8879, 594.378) ccw
  arc A284 (475, 520.4805) -> (475, 525.4754) centre (474.8879, 522.978) ccw
  arc A285 (475, 551.0805) -> (475, 556.0754) centre (474.8879, 553.578) ccw
  line L211 (475, 505.0754) -> (475, 505.1805)
  circle A286 centre (545, 423.2517) radius 12.5
  line L212 (551.3824, 597.2378) -> (598.9426, 502.2076)
  line L213 (550, 445) -> (550, 446.5033)
  line L214 (500, 445) -> (500, 400) construction
  line L215 (475, 300) -> (475, 250) construction
  line L216 (395, 250) -> (395, 300) construction
  arc A287 (525, 550.9754) -> (525, 545.9805) centre (524.8879, 548.478) ccw
  line L217 (395, 300) -> (400, 300) construction
  line L218 (400, 300) -> (425, 250) construction
  line L219 (400, 300) -> (450, 300)
  arc A288 (550, 446.5033) -> (548.9884, 450.8862) centre (540, 446.5033) ccw
  arc A289 (451.0557, 452.1115) -> (450, 447.6393) centre (460, 447.6393) ccw
  circle A290 centre (455, 425) radius 12.5
  line L220 (450, 445) -> (450, 447.6393)
  line L221 (450, 400) -> (470, 400)
  line L222 (450, 445) -> (470, 445)
  line L223 (550, 400) -> (530, 400)
  line L224 (550, 445) -> (530, 445)
  line L225 (470, 400) -> (475, 400)
  line L226 (475, 445) -> (475, 400)
  line L227 (475, 445) -> (470, 445)
  line L228 (530, 400) -> (525, 400)
  line L229 (525, 400) -> (525, 445)
  line L230 (530, 445) -> (525, 445)
  line L231 (455, 425) -> (475, 425) construction
  line L232 (545, 423.2517) -> (525, 423.2517) construction
  line L233 (1580, 550) -> (1320, 550)
  line L234 (1300, 400) -> (1300, 600)
  line L235 (1300, 600) -> (1600, 600)
  line L236 (1320, 550) -> (1320, 580)
  line L237 (1320, 580) -> (1580, 580)
  line L238 (1600, 600) -> (1600, 400)
  line L239 (1580, 580) -> (1580, 550)
  line L240 (1600, 400) -> (1300, 400)
  point P0 (175, 595)
  point P1 (175, 503.541)
  point P2 (175, 503.541)
  point P3 (525, 595)
  point P4 (525, 503.541)
  point P5 (525, 503.541)
  dimension "d29" = 360
  dimension "d40" = 10
  dimension "d44" = 25
  dimension "d45" = 10
  dimension "d46" = 10
  dimension "d47" = 10
  dimension "d48" = 15
  dimension "d49" = 25
  dimension "d51" = 10
  dimension "d52" = 15
  dimension "d53" = 5
  dimension "d54" = 5
  dimension "d55" = 5
  dimension "d56" = 10
  dimension "d57" = 25
  dimension "d58" = 5
  dimension "d59" = 5
  dimension "d60" = 5
  dimension "d61" = 5
  dimension "d62" = 5
  dimension "d63" = 5
  dimension "d64" = 5
  dimension "d65" = 5
  dimension "d66" = 5
  dimension "d67" = 5
  dimension "d68" = 5
  dimension "d69" = 5
  dimension "d70" = 5
  dimension "d71" = 5
  dimension "d72" = 5
  dimension "d73" = 5
  dimension "d74" = 5
  dimension "d75" = 5
  dimension "d76" = 5
  dimension "d79" = 5
  dimension "d80" = 5
  dimension "d81" = 5
  dimension "d82" = 5
  dimension "d83" = 5
  dimension "d84" = 5
  dimension "d85" = 5
  dimension "d86" = 5
  dimension "d87" = 5
  dimension "d88" = 5
  dimension "d89" = 5
  dimension "d90" = 5
  dimension "d91" = 5
  dimension "d92" = 5
  dimension "d93" = 5
  dimension "d94" = 5
  dimension "d95" = 5
  dimension "d96" = 5
  dimension "d97" = 5
  dimension "d101" = 25
  dimension "d102" = 25
  dimension "d113" = 25
  dimension "d114" = 21
  dimension "d122" = 300
  dimension "d123" = 200
  dimension "d127" = 360
  dimension "d135" = 10
  dimension "d137" = 10
  dimension "d138" = 10
  dimension "d139" = 10
  dimension "d140" = 15
  dimension "d141" = 25
  dimension "d142" = 10
  dimension "d143" = 15
  dimension "d144" = 5
  dimension "d145" = 5
  dimension "d146" = 5
  dimension "d147" = 10
  dimension "d148" = 25
  dimension "d149" = 5
  dimension "d150" = 5
  dimension "d151" = 5
  dimension "d152" = 5
  dimension "d153" = 5
  dimension "d154" = 5
  dimension "d155" = 5
  dimension "d156" = 5
  dimension "d157" = 5
  dimension "d158" = 5
  dimension "d159" = 5
  dimension "d160" = 5
  dimension "d161" = 5
  dimension "d162" = 5
  dimension "d163" = 5
  dimension "d164" = 5
  dimension "d165" = 5
  dimension "d166" = 5
  dimension "d167" = 5
  dimension "d168" = 5
  dimension "d169" = 5
  dimension "d170" = 5
  dimension "d171" = 5
  dimension "d172" = 5
  dimension "d173" = 5
  dimension "d174" = 5
  dimension "d175" = 5
  dimension "d176" = 5
  dimension "d177" = 5
  dimension "d178" = 5
  dimension "d179" = 5
  dimension "d180" = 5
  dimension "d181" = 5
  dimension "d182" = 5
  dimension "d183" = 5
  dimension "d184" = 5
  dimension "d185" = 5
  dimension "d186" = 5
  dimension "d187" = 25
  dimension "d188" = 25
  dimension "d189" = 25
  dimension "d190" = 100
  dimension "d191" = 20
  dimension "d206" = 300
  dimension "d207" = 200
  constraint horizontal L0
  constraint vertical L30
  constraint horizontal L1
  constraint vertical L2
  constraint horizontal L3
  constraint vertical L4
  constraint horizontal L5
  constraint vertical L28
  constraint midpoint L1 L13.start
  constraint perpendicular L2 L10
  constraint perpendicular L12 L30
  constraint midpoint L13 L6.start
  constraint perpendicular L4 L22
  constraint perpendicular L4 L24
  constraint collinear L28 L29
  constraint perpendicular L1 L31
  constraint perpendicular L31 L32
  constraint perpendicular L5 L33
  constraint perpendicular L33 L34
  constraint perpendicular L5 L35
  constraint perpendicular L0 L36
  constraint perpendicular L36 L37
  constraint perpendicular L37 L38
  constraint perpendicular L39 L40
  constraint perpendicular L1 L41
  constraint coincident L2 L10.start
  constraint collinear L44 L45
  constraint concentric A1 A79
  constraint concentric A72 A88
  constraint concentric A73 A74
  constraint concentric A74 A75
  constraint concentric A75 A76
  constraint concentric A76 A77
  constraint concentric A77 A78
  constraint concentric A78 A79
  constraint concentric A79 A80
  constraint concentric A80 A81
  constraint concentric A81 A82
  constraint concentric A82 A83
  constraint concentric A83 A84
  constraint concentric A84 A85
  constraint concentric A85 A86
  constraint concentric A86 A87
  constraint concentric A87 A89
  constraint concentric A88 A89
  constraint perpendicular L46 L61
  constraint tangent L46 A91
  constraint perpendicular L52 L60
  constraint tangent A94 L50
  constraint tangent A94 L52
  constraint tangent A93 L50
  constraint tangent L47 A93
  constraint tangent L51 A96
  constraint tangent L49 A96
  constraint tangent A95 L59
  constraint tangent L49 A95
  constraint vertical L53
  constraint tangent L54 A98
  constraint tangent L55 A98
  constraint tangent L55 A99
  constraint tangent A99 L94
  constraint tangent A100 L111
  constraint tangent L56 A100
  constraint tangent A101 L61
  constraint tangent L46 A101
  constraint tangent L56 A102
  constraint tangent L57 A102
  constraint tangent L53 A103
  constraint tangent L57 A103
  constraint collinear L58 L62
  constraint collinear L59 L64
  constraint collinear L63 L66
  constraint collinear L65 L68
  constraint collinear L67 L72
  constraint collinear L69 L70
  constraint collinear L71 L76
  constraint collinear L73 L74
  constraint collinear L77 L80
  constraint collinear L75 L78
  constraint collinear L81 L82
  constraint collinear L79 L84
  constraint collinear L83 L88
  constraint collinear L85 L86
  constraint collinear L89 L92
  constraint collinear L87 L90
  constraint collinear L60 L93
  constraint collinear L61 L91
  constraint collinear L95 L96
  constraint collinear L97 L98
  constraint collinear L99 L100
  constraint collinear L101 L102
  constraint collinear L103 L104
  constraint collinear L105 L106
  constraint collinear L107 L108
  constraint collinear L109 L110
  constraint collinear L62 L63
  constraint collinear L64 L65
  constraint collinear L66 L67
  constraint collinear L68 L69
  constraint collinear L70 L71
  constraint collinear L72 L73
  constraint collinear L74 L75
  constraint collinear L76 L77
  constraint collinear L78 L79
  constraint collinear L80 L81
  constraint collinear L82 L83
  constraint collinear L84 L85
  constraint collinear L86 L87
  constraint collinear L88 L89
  constraint collinear L90 L91
  constraint collinear L92 L93
  constraint collinear L94 L95
  constraint collinear L96 L97
  constraint collinear L98 L99
  constraint collinear L100 L101
  constraint collinear L102 L103
  constraint collinear L104 L105
  constraint collinear L106 L107
  constraint collinear L108 L109
  constraint collinear L110 L111
  constraint perpendicular L112 L113
  constraint perpendicular L115 L116
  constraint perpendicular L114 L118
  constraint perpendicular L118 L119
  constraint perpendicular L119 L120
  constraint perpendicular L113 L121
  constraint perpendicular L112 L122
  constraint coincident L120 L124.end
  constraint parallel L123 L124
  constraint horizontal L125
  constraint vertical L126
  constraint horizontal L127
  constraint vertical L128
  constraint horizontal L129
  constraint vertical L130
  constraint horizontal L131
  constraint vertical L132
  constraint horizontal L133
  constraint vertical L134
  constraint horizontal L135
  constraint vertical L136
  constraint concentric A205 A209
  constraint concentric A208 A230
  constraint concentric A188 A234
  constraint concentric A188 A224
  constraint concentric A211 A224
  constraint concentric A201 A211
  constraint concentric A150 A201
  constraint concentric A150 A209
  constraint concentric A209 A212
  constraint concentric A212 A217
  constraint concentric A183 A217
  constraint concentric A164 A183
  constraint concentric A164 A207
  constraint concentric A173 A207
  constraint concentric A170 A173
  constraint concentric A158 A170
  constraint concentric A158 A218
  constraint concentric A208 A218
  constraint coincident L51 L137.start
  constraint coincident L54 L137.end
  constraint perpendicular L54 L137
  constraint perpendicular L115 L138
  constraint midpoint L137 L139.start
  constraint midpoint L138 L139.end
  constraint perpendicular L180 L200
  constraint tangent A262 L180
  constraint perpendicular L151 L174
  constraint tangent A250 L161
  constraint tangent A250 L174
  constraint tangent A241 L161
  constraint tangent A241 L183
  constraint tangent A289 L220
  constraint tangent L181 A289
  constraint tangent A273 L211
  constraint tangent L181 A273
  constraint vertical L143
  constraint tangent L213 A288
  constraint tangent L184 A288
  constraint tangent A247 L184
  constraint tangent A247 L175
  constraint tangent A244 L188
  constraint tangent A244 L195
  constraint tangent A279 L200
  constraint tangent L180 A279
  constraint tangent A251 L195
  constraint tangent A251 L212
  constraint tangent A238 L143
  constraint tangent A238 L212
  constraint collinear L150 L156
  constraint collinear L193 L211
  constraint collinear L160 L205
  constraint collinear L155 L198
  constraint collinear L187 L209
  constraint collinear L154 L191
  constraint collinear L177 L197
  constraint collinear L163 L189
  constraint collinear L147 L159
  constraint collinear L153 L192
  constraint collinear L196 L202
  constraint collinear L186 L201
  constraint collinear L204 L206
  constraint collinear L158 L203
  constraint collinear L194 L207
  constraint collinear L179 L210
  constraint collinear L151 L199
  constraint collinear L200 L208
  constraint collinear L148 L171
  constraint collinear L149 L152
  constraint collinear L157 L162
  constraint collinear L146 L164
  constraint collinear L167 L176
  constraint collinear L172 L178
  constraint collinear L145 L170
  constraint collinear L144 L190
  constraint collinear L156 L160
  constraint collinear L193 L198
  constraint collinear L205 L209
  constraint collinear L155 L191
  constraint collinear L154 L197
  constraint collinear L163 L187
  constraint collinear L153 L189
  constraint collinear L159 L177
  constraint collinear L186 L192
  constraint collinear L147 L196
  constraint collinear L202 L206
  constraint collinear L201 L203
  constraint collinear L158 L210
  constraint collinear L194 L204
  constraint collinear L179 L208
  constraint collinear L199 L207
  constraint collinear L148 L175
  constraint collinear L149 L171
  constraint collinear L152 L162
  constraint collinear L157 L164
  constraint collinear L146 L176
  constraint collinear L167 L172
  constraint collinear L170 L178
  constraint collinear L144 L145
  constraint collinear L188 L190
  constraint perpendicular L165 L219
  constraint perpendicular L173 L182
  constraint perpendicular L166 L169
  constraint perpendicular L169 L215
  constraint perpendicular L216 L219
  constraint perpendicular L165 L217
  constraint parallel L168 L218
  constraint perpendicular L185 L213
  constraint perpendicular L141 L173
  constraint midpoint L214.start L185
  constraint midpoint L214.end L141
  constraint coincident L141 L221.end
  constraint perpendicular L220 L221
  constraint coincident L185 L222.end
  constraint coincident L141 L223.end
  constraint perpendicular L213 L223
  constraint coincident L185 L224.end
  constraint coincident L141 L225.end
  constraint coincident L185 L226.start
  constraint perpendicular L141 L226
  constraint coincident L141 L228.end
  constraint coincident L185 L229.end
  constraint perpendicular L185 L229
  constraint coincident A290.centre L231.start
  constraint coincident L226 L231.end
  constraint perpendicular L226 L231
  constraint coincident A286.centre L232.start
  constraint coincident L229 L232.end
  constraint perpendicular L229 L232
  constraint horizontal L235
  constraint vertical L238
  constraint horizontal L240
  constraint vertical L234
  constraint horizontal L237
  constraint vertical L239
  constraint horizontal L233
  constraint vertical L236
  measures "d40" radius of A91
  measures "d44" diameter of A92
  measures "d45" radius of A94
  measures "d46" radius of A93
  measures "d47" radius of A96
  measures "d48" radius of A95
  measures "d49" diameter of A97
  measures "d51" radius of A98
  measures "d52" radius of A99
  measures "d53" radius of A100
  measures "d54" radius of A101
  measures "d55" radius of A102
  measures "d56" radius of A103
  measures "d57" diameter of A104
  measures "d58" diameter of A123
  measures "d59" diameter of A105
  measures "d60" diameter of A124
  measures "d61" diameter of A106
  measures "d62" diameter of A125
  measures "d63" diameter of A107
  measures "d64" diameter of A126
  measures "d65" diameter of A108
  measures "d66" diameter of A127
  measures "d67" diameter of A109
  measures "d68" diameter of A128
  measures "d69" diameter of A110
  measures "d70" diameter of A129
  measures "d71" diameter of A111
  measures "d72" diameter of A130
  measures "d73" diameter of A112
  measures "d74" diameter of A131
  measures "d75" diameter of A113
  measures "d76" diameter of A132
  measures "d79" diameter of A133
  measures "d80" diameter of A114
  measures "d81" diameter of A134
  measures "d82" diameter of A115
  measures "d83" diameter of A135
  measures "d84" diameter of A116
  measures "d85" diameter of A136
  measures "d86" diameter of A117
  measures "d87" diameter of A137
  measures "d88" diameter of A118
  measures "d89" diameter of A138
  measures "d90" diameter of A119
  measures "d91" diameter of A139
  measures "d92" diameter of A120
  measures "d93" diameter of A140
  measures "d94" diameter of A121
  measures "d95" diameter of A141
  measures "d96" diameter of A122
  measures "d97" diameter of A142
  measures "d101" diameter of A143
  measures "d102" diameter of A144
  measures "d113" diameter of A143
  measures "d114" diameter of A146
  measures "d122" distance of L126.end L127.end
  measures "d123" distance of L125.end L126.end
  measures "d135" radius of A262
  measures "d137" radius of A250
  measures "d138" radius of A241 A21.end
  measures "d139" radius of A289
  measures "d140" radius of A273
  measures "d141" diameter of A290
  measures "d142" radius of A288
  measures "d143" radius of A247
  measures "d144" radius of A244
  measures "d145" radius of A279
  measures "d146" radius of A251
  measures "d147" radius of A238
  measures "d148" diameter of A286
  measures "d149" diameter of A266
  measures "d150" diameter of A254
  measures "d151" diameter of A243
  measures "d152" diameter of A246
  measures "d153" diameter of A284
  measures "d154" diameter of A276
  measures "d155" diameter of A272
  measures "d156" diameter of A242
  measures "d157" diameter of A268
  measures "d158" diameter of A253
  measures "d159" diameter of A285
  measures "d160" diameter of A274
  measures "d161" diameter of A275
  measures "d162" diameter of A280
  measures "d163" diameter of A278
  measures "d164" diameter of A271
  measures "d165" diameter of A282
  measures "d166" diameter of A281
  measures "d167" diameter of A283
  measures "d168" diameter of A248
  measures "d169" diameter of A261
  measures "d170" diameter of A240
  measures "d171" diameter of A259
  measures "d172" diameter of A258
  measures "d173" diameter of A263
  measures "d174" diameter of A256
  measures "d175" diameter of A252
  measures "d176" diameter of A287
  measures "d177" diameter of A265
  measures "d178" diameter of A257
  measures "d179" diameter of A267
  measures "d180" diameter of A264
  measures "d181" diameter of A260
  measures "d182" diameter of A239
  measures "d183" diameter of A255
  measures "d184" diameter of A249
  measures "d185" diameter of A277
  measures "d186" diameter of A245
  measures "d187" diameter of A270
  measures "d188" diameter of A269
  measures "d189" diameter of A270
  measures "d190" distance of L141.start L141.end
  measures "d191" distance of L141.start L221.end
  measures "d206" distance of L234.start L238.end
  measures "d207" distance of L235.end L238.end